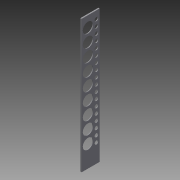
# Autodesk Inventor part: speakerfront
Saved by Autodesk Inventor 2015 (Build 190159000, 159)
## iProperties
Created: 2015-02-03
Part Number: speakerfront
Material: Generic
Document SubType Name: Modeling
Designer: rubidium
Density: 1 g/cm^3
Appearance: Default
Author: rubidium
Autodesk Inventor part; units mm, degrees
ref_plane "YZ Plane" through (0, 0, 0) normal (1, 0, 0) x (0, 1, 0)
ref_plane "XZ Plane" through (0, 0, 0) normal (0, 1, 0) x (-1, 0, 0)
ref_plane "XY Plane" through (0, 0, 0) normal (0, 0, 1) x (1, 0, 0)
sketch "Sketch1" plane through (0, 0, 0) normal (1, 0, 0) x (0, 1, 0)
  line L0 (1109.5249, 0) -> (-770.0751, 0)
  line L1 (-770.0751, 0) -> (-770.0751, -254)
  line L2 (-770.0751, -254) -> (1109.5249, -254)
  line L3 (1109.5249, -254) -> (1109.5249, 0)
  circle A0 centre (-465.2751, -88.9) radius 73.025
  circle A1 centre (-509.7251, -209.55) radius 25.4
  circle A2 centre (-420.8251, -209.55) radius 25.4
  circle A3 centre (-287.4751, -88.9) radius 73.025
  circle A4 centre (-331.9251, -209.55) radius 25.4
  circle A5 centre (-243.0251, -209.55) radius 25.4
  circle A6 centre (-109.6751, -88.9) radius 73.025
  circle A7 centre (-154.1251, -209.55) radius 25.4
  circle A8 centre (-65.2251, -209.55) radius 25.4
  circle A9 centre (68.1249, -88.9) radius 73.025
  circle A10 centre (23.6749, -209.55) radius 25.4
  circle A11 centre (112.5749, -209.55) radius 25.4
  circle A12 centre (245.9249, -88.9) radius 73.025
  circle A13 centre (201.4749, -209.55) radius 25.4
  circle A14 centre (290.3749, -209.55) radius 25.4
  circle A15 centre (423.7249, -88.9) radius 73.025
  circle A16 centre (379.2749, -209.55) radius 25.4
  circle A17 centre (468.1749, -209.55) radius 25.4
  circle A18 centre (601.5249, -88.9) radius 73.025
  circle A19 centre (557.0749, -209.55) radius 25.4
  circle A20 centre (645.9749, -209.55) radius 25.4
  circle A21 centre (779.3249, -88.9) radius 73.025
  circle A22 centre (734.8749, -209.55) radius 25.4
  circle A23 centre (823.7749, -209.55) radius 25.4
  circle A24 centre (957.1249, -88.9) radius 73.025
  circle A25 centre (912.6749, -209.55) radius 25.4
  circle A26 centre (1001.5749, -209.55) radius 25.4
  point P0 (0, 0)
  point P1 (-163.267, 0)
  dimension "d0" = 254
  dimension "d1" = 1879.6
  dimension "d10" = 146.05
  dimension "d16" = 50.8
  dimension "d20" = 304.8
  dimension "d21" = 44.45
  dimension "d22" = 120.65
  dimension "d24" = 88.9
  dimension "d25" = 50.8
  dimension "d26" = 88.9
  dimension "d27" = 120.65
  dimension "d30" = 177.8
  constraints: 27 centre point, 8 end point, 2 horizontal, 2 parallel, 1 perpendicular, 48 other
  measures "d0" distance of L0.end L1.end
  measures "d1" distance of L1.end L2.end
  measures "d10" diameter of A0
  measures "d16" diameter of A1
  measures "d20" horizontal distance of L0.end A0.centre
  measures "d21" horizontal distance of A0.centre A1.centre
  measures "d22" vertical distance of A0.centre A1.centre
  measures "d24" distance from line of L0 A0.centre
  measures "d25" diameter of A2
  measures "d26" distance of A2.centre A1.centre
  measures "d27" vertical distance of A0.centre A2.centre
  measures "d30" distance of A0.centre A3.centre
extrude "Extrusion1" add sketch "Sketch1" along normal blind 17.78
fillet "Fillet1" radius 12.7 27 edges at (0, 884.0999, -88.9) (0, 706.2999, -88.9) (0, 528.4999, -88.9) (0, 350.6999, -88.9) (0, 172.8999, -88.9) (0, -4.9001, -88.9) (0, -182.7001, -88.9) (0, -360.5001, -88.9) (0, -538.3001, -88.9) (0, -357.3251, -209.55) (0, -446.2251, -209.55) (0, -535.1251, -209.55) (0, -268.4251, -209.55) (0, -179.5251, -209.55) (0, -90.6251, -209.55) (0, -1.7251, -209.55) (0, 87.1749, -209.55) (0, 176.0749, -209.55) (0, 264.9749, -209.55) (0, 353.8749, -209.55) (0, 442.7749, -209.55) (0, 531.6749, -209.55) (0, 620.5749, -209.55) (0, 709.4749, -209.55) (0, 798.3749, -209.55) (0, 887.2749, -209.55) (0, 976.1749, -209.55)
body "Solid1"
